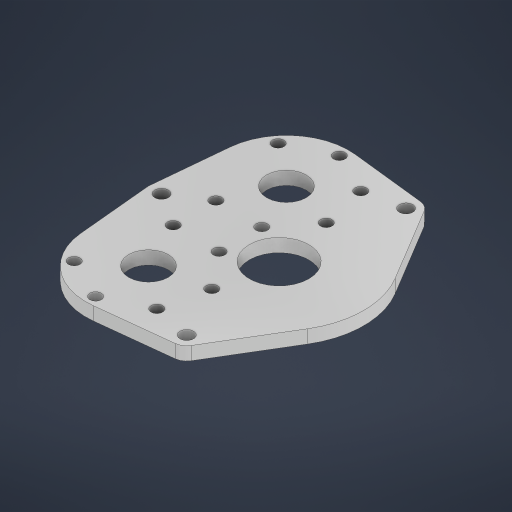
# Autodesk Inventor part: Part1
Saved by Autodesk Inventor 2024.3 (Build 283343000, 343)
## iProperties
Created: 2024-10-27
Part Number: Part1
Material: Aluminum 6061
Document SubType Name: Modeling
Designer: kaito
Mass: 153.708 g
Surface Area: 233.757 cm^2
Volume: 56.9288 cm^3
Density: 2.7 g/cm^3
Appearance: Aluminum - Polished
Author: kaito
Autodesk Inventor part; units mm, degrees
ref_plane "YZ Plane" through (0, 0, 0) normal (1, 0, 0) x (0, 1, 0)
ref_plane "XZ Plane" through (0, 0, 0) normal (0, 1, 0) x (-1, 0, 0)
ref_plane "XY Plane" through (0, 0, 0) normal (0, 0, 1) x (1, 0, 0)
sketch "Sketch1" plane through (0, 0, 0) normal (0, 1, 0) x (-1, 0, 0)
  circle A0 centre (29.6155, 33.147) radius 6.35 construction
  circle A1 centre (0, 0) radius 38.1 construction
  circle A2 centre (29.6155, -33.147) radius 6.35 construction
  circle A3 centre (29.6155, 33.147) radius 29.972 construction
  circle A4 centre (29.6155, -33.147) radius 29.972 construction
  line L0 (29.6155, 3.175) -> (29.6155, -3.175) construction
  circle A5 centre (0, 0) radius 40.64 construction
  circle A6 centre (-8.3197, 52.6872) radius 6.35 construction
  circle A7 centre (-8.3197, 52.6872) radius 3.2639
  line L1 (-7.3293, 46.4149) -> (-6.3388, 40.1426) construction
  line L2 (-2.6746, 49.7794) -> (2.9705, 46.8716) construction
  circle A8 centre (-8.3197, -52.6872) radius 6.35 construction
  circle A9 centre (-8.3197, -52.6872) radius 3.2639
  line L3 (-7.3293, -46.4149) -> (-6.3388, -40.1426) construction
  line L4 (2.9705, -46.8716) -> (-2.6746, -49.7794) construction
  circle A10 centre (56.4888, 0) radius 6.35 construction
  circle A11 centre (56.4888, 0) radius 3.2639
  line L5 (48.4908, 9.8652) -> (52.4898, 4.9326) construction
  line L6 (52.4898, -4.9326) -> (48.4908, -9.8652) construction
  circle A12 centre (0, 0) radius 14.2875
  circle A13 centre (29.6155, 33.147) radius 9.525
  circle A14 centre (29.6155, -33.147) radius 9.525
  circle A15 centre (29.6155, 33.147) radius 25.4 construction
  circle A16 centre (29.6155, 58.547) radius 2.794
  circle A17 centre (49.474, 48.9836) radius 2.794
  circle A18 centre (54.3787, 27.495) radius 2.794 construction
  circle A19 centre (40.6362, 10.2624) radius 2.794
  circle A20 centre (18.5949, 10.2624) radius 2.794
  circle A21 centre (4.8523, 27.495) radius 2.794
  circle A22 centre (9.757, 48.9836) radius 2.794
  circle A23 centre (29.6155, -33.147) radius 25.4 construction
  circle A24 centre (29.6155, -58.547) radius 2.794
  circle A25 centre (49.474, -48.9836) radius 2.794
  circle A26 centre (54.3787, -27.495) radius 2.794 construction
  circle A27 centre (40.6362, -10.2624) radius 2.794
  circle A28 centre (18.5949, -10.2624) radius 2.794
  circle A29 centre (4.8523, -27.495) radius 2.794
  circle A30 centre (9.757, -48.9836) radius 2.794
  line L7 (26.2955, 62.9346) -> (-9.0231, 58.9981)
  line L8 (-13.7609, 55.9607) -> (-34.8236, 20.9505)
  line L9 (-34.8236, -20.9505) -> (-13.7609, -55.9607)
  line L10 (-9.0231, -58.9981) -> (26.2955, -62.9346)
  line L11 (59.4535, -35.9782) -> (62.8105, -0.5998)
  line L12 (62.8105, 0.5998) -> (59.4535, 35.9782)
  arc A31 (-9.0231, 58.9981) -> (-13.7609, 55.9607) centre (-8.3197, 52.6872) ccw
  arc A32 (59.4535, 35.9782) -> (26.2955, 62.9346) centre (29.6155, 33.147) ccw
  arc A33 (-34.8236, 20.9505) -> (-34.8236, -20.9505) centre (0, 0) ccw
  arc A34 (-13.7609, -55.9607) -> (-9.0231, -58.9981) centre (-8.3197, -52.6872) ccw
  arc A35 (26.2955, -62.9346) -> (59.4535, -35.9782) centre (29.6155, -33.147) ccw
  arc A36 (62.8105, -0.5998) -> (62.8105, 0.5998) centre (56.4888, 0) ccw
  point P0 (29.6155, 0)
  dimension "d21" = 50.8
  dimension "d27" = 50.8
  dimension "d0" = 12.7
  dimension "d1" = 76.2
  dimension "d2" = 12.7
  dimension "d3" = 59.944
  dimension "d4" = 59.944
  dimension "d5" = 6.35
  dimension "d6" = 2.54
  dimension "d8" = 12.7
  dimension "d9" = 6.5278
  dimension "d11" = 6.35
  dimension "d12" = 12.7
  dimension "d13" = 6.5278
  dimension "d14" = 6.35
  dimension "d15" = 12.7
  dimension "d16" = 6.5278
  dimension "d17" = 6.35
  dimension "d18" = 6.35
  dimension "d19" = 28.575
  dimension "d20" = 19.05
  dimension "d22" = 5.588
  dimension "d25" = 360
  dimension "d30" = 360
  constraints: 39 point on circle, 35 centre point, 26 end point, 17 tangent, 14 point on line, 10 coincident, 7 equal radius, 4 vertical alignment, 2 equal length, 1 horizontal alignment, 1 midpoint, 34 other
  measures "d0" diameter of A0
  measures "d1" diameter of A1
  measures "d2" diameter of A2
  measures "d3" diameter of A3
  measures "d4" diameter of A4
  measures "d5" distance of L0.start L0.end
  measures "d6" radial gap between concentric circles of A1 A5
  measures "d8" diameter of A6
  measures "d9" diameter of A7
  measures "d11" distance of L1.start L1.end
  measures "d12" diameter of A8
  measures "d13" diameter of A9
  measures "d14" distance of L3.start L3.end
  measures "d15" diameter of A10
  measures "d16" diameter of A11
  measures "d17" distance of L5.start L5.end
  measures "d18" distance of L6.start L6.end
  measures "d19" diameter of A12
  measures "d20" diameter of A13
  measures "d22" diameter of A16
extrude "Extrusion1" add sketch "Sketch1" along normal blind 6.35
body "Solid1"
